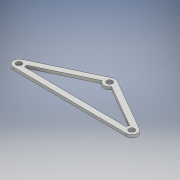
# Autodesk Inventor part: 三角塊2
Saved by Autodesk Inventor 2017 (Build 210142000, 142)
## iProperties
Part Number: 三角塊2
Material: 一般
Document SubType Name: Modeling
Designer: user
Density: 1 g/cm^3
Appearance: 預設
Author: user
Autodesk Inventor part; units mm, degrees
ref_plane "YZ Plane" through (0, 0, 0) normal (1, 0, 0) x (0, 1, 0)
ref_plane "XZ Plane" through (0, 0, 0) normal (0, 1, 0) x (-1, 0, 0)
ref_plane "XY Plane" through (0, 0, 0) normal (0, 0, 1) x (1, 0, 0)
sketch "草圖1" plane through (0, 0, 0) normal (0, 0, 1) x (1, 0, 0)
  line L0 (-1.7305, 1.0027) -> (-17.0365, 9.8719)
  line L1 (-18.7669, 10.8747) -> (-38.873, 1.2756)
  line L2 (-40.6779, 0.4139) -> (-1.9999, 0.0203)
  line L3 (8.4583, -2.0862) -> (-44.617, -1.5461)
  line L4 (-19.6286, 12.6795) -> (-43.3233, 1.3672)
  line L5 (7.8765, -2.2526) -> (-17.7642, 12.6051)
  arc A0 (-17.7642, 12.6051) -> (-19.6286, 12.6795) centre (-18.7669, 10.8747) ccw
  arc A1 (-20.5718, 10.013) -> (-17.0365, 9.8719) centre (-18.7669, 10.8747) ccw
  arc A2 (-1.7305, 1.0027) -> (-1.9999, 0.0203) centre (0, 0) ccw
  arc A3 (-0.0203, -1.9999) -> (1.0027, 1.7305) centre (0, 0) ccw
  arc A4 (-41.5396, 2.2188) -> (-40.6982, -1.586) centre (-40.6779, 0.4139) ccw
  arc A5 (-38.678, 0.3936) -> (-38.873, 1.2756) centre (-40.6779, 0.4139) ccw
  dimension "d0" = 21.69
  dimension "d1" = 24.28
  dimension "d2" = 40.68
  constraints: 12 end point, 12 point on circle, 6 centre point, 6 point on line, 6 tangent, 3 coincident
  measures "d0" distance of point (0, 0) L1.start
  measures "d1" distance of L1.start L2.start
  measures "d2" distance of L2.start point (0, 0)
extrude "擠出1" add sketch "草圖1" along normal blind 1 contours L3 A4 L4 A0 L5 A3
sketch "草圖2" plane through (0, 0, 1) normal (0, 0, 1) x (1, 0, 0)
  arc A0 (-20.5718, 10.013) -> (-17.0365, 9.8719) centre (-18.7669, 10.8747) ccw projected
  circle A1 centre (-18.7669, 10.8747) radius 1
  circle A2 centre (0, 0) radius 1
  arc A3 (-38.678, 0.3936) -> (-38.873, 1.2756) centre (-40.6779, 0.4139) ccw projected
  circle A4 centre (-40.6779, 0.4139) radius 1
  dimension "d8" = 2
  dimension "d9" = 2
  dimension "d10" = 2
  constraints: 3 centre point, 3 coincident
  measures "d8" diameter of A1
  measures "d9" diameter of A2
  measures "d10" diameter of A4
extrude "擠出2" cut sketch "草圖2" against normal blind 10
